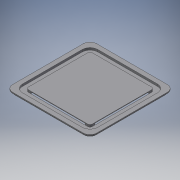
# Autodesk Inventor part: NewLid
Saved by Autodesk Inventor 2017 (Build 210142000, 142)
## iProperties
Created: 2019-11-20
Part Number: NewLid
Material: Generic
Document SubType Name: Modeling
Designer: DDeGo
Density: 1 g/cm^3
Appearance: Default
Author: DDeGo
Autodesk Inventor part; units mm, degrees
ref_plane "YZ Plane" through (0, 0, 0) normal (1, 0, 0) x (0, 1, 0)
ref_plane "XZ Plane" through (0, 0, 0) normal (0, 1, 0) x (-1, 0, 0)
ref_plane "XY Plane" through (0, 0, 0) normal (0, 0, 1) x (1, 0, 0)
sketch "Sketch1" plane through (0, 0, 0) normal (0, 0, 1) x (1, 0, 0)
  arc A0 (-15, -160) -> (0, -175) centre (0, -160) ccw
  line L0 (0, 15) -> (160, 15)
  line L1 (175, 0) -> (175, -160)
  line L2 (160, -175) -> (0, -175)
  line L3 (-15, -160) -> (-15, 0)
  arc A1 (0, 15) -> (-15, 0) centre (0, 0) ccw
  arc A2 (160, -175) -> (175, -160) centre (160, -160) ccw
  arc A3 (175, 0) -> (160, 15) centre (160, 0) ccw
  point P0 (-15, 15)
  dimension "d0" = 190
  dimension "d1" = 190
  dimension "d2" = 15
  constraints: 8 end point, 8 point on circle, 8 tangent, 4 centre point, 3 equal radius, 2 coincident, 2 parallel, 2 point on line, 1 horizontal, 1 perpendicular
  measures "d0" distance between parallel lines of L2 L0
  measures "d1" distance between parallel lines of L3 L1
  measures "d2" radius of A3
extrude "Extrusion1" add sketch "Sketch1" along normal blind 6.35
sketch "Sketch2" plane through (0, 0, 6.35) normal (0, 0, 1) x (1, 0, 0)
  line L0 (-15, 0) -> (-15, -160) projected
  arc A0 (-15, -160) -> (0, -175) centre (0, -160) ccw projected
  line L1 (0, -175) -> (160, -175) projected
  arc A1 (160, -175) -> (175, -160) centre (160, -160) ccw projected
  line L2 (175, -160) -> (175, 0) projected
  arc A2 (175, 0) -> (160, 15) centre (160, 0) ccw projected
  line L3 (160, 15) -> (0, 15) projected
  arc A3 (0, 15) -> (-15, 0) centre (0, 0) ccw projected
  line L4 (0, 0) -> (160, -160) construction
  line L5 (147.3, -152.3) -> (12.7, -152.3)
  line L6 (7.7, -147.3) -> (7.7, -12.7)
  line L7 (12.7, -7.7) -> (147.3, -7.7)
  line L8 (152.3, -12.7) -> (152.3, -147.3)
  line L9 (152.3, -152.3) -> (7.7, -7.7) construction
  line L10 (7.7, -152.3) -> (152.3, -7.7) construction
  arc A4 (12.7, -7.7) -> (7.7, -12.7) centre (12.7, -12.7) ccw
  arc A5 (152.3, -12.7) -> (147.3, -7.7) centre (147.3, -12.7) ccw
  arc A6 (147.3, -152.3) -> (152.3, -147.3) centre (147.3, -147.3) ccw
  arc A7 (7.7, -147.3) -> (12.7, -152.3) centre (12.7, -147.3) ccw
  line L11 (147.3, 5) -> (12.7, 5)
  arc A8 (12.7, 5) -> (-5, -12.7) centre (12.7, -12.7) ccw
  line L12 (-5, -12.7) -> (-5, -147.3)
  arc A9 (-5, -147.3) -> (12.7, -165) centre (12.7, -147.3) ccw
  line L13 (12.7, -165) -> (147.3, -165)
  arc A10 (147.3, -165) -> (165, -147.3) centre (147.3, -147.3) ccw
  line L14 (165, -147.3) -> (165, -12.7)
  arc A11 (165, -12.7) -> (147.3, 5) centre (147.3, -12.7) ccw
  point P0 (80, -80)
  dimension "d7" = 5
  dimension "d8" = 12.7
  dimension "d9" = 10
  constraints: 22 end point, 16 point on circle, 9 point on line, 8 centre point, 8 tangent, 4 parallel, 3 equal radius, 3 midpoint, 2 perpendicular, 1 horizontal, 7 other
  measures "d7" radius of A4
  measures "d8" distance between parallel lines of L7 L11
  measures "d9" distance between parallel lines of L2 L14
extrude "Extrusion2" cut sketch "Sketch2" against normal blind 5 contours A11 L14 A10 L13 A9 L12 A8 L11
sketch "Sketch3" plane through (0, 0, 0) normal (0, 0, -1) x (-1, 0, 0)
  line L0 (-140, -10.675) -> (-20, -10.675) construction
  line L1 (-147.3, -7.7) -> (-12.7, -7.7) projected
  line L2 (-140, -13.85) -> (-20, -13.85)
  line L3 (-20, -7.5) -> (-140, -7.5)
  arc A0 (-140, -7.5) -> (-140, -13.85) centre (-140, -10.675) ccw
  arc A1 (-20, -13.85) -> (-20, -7.5) centre (-20, -10.675) ccw
  line L4 (15, -160) -> (15, 0) projected
  line L5 (-175, 0) -> (-175, -160) projected
  arc A2 (-160, 15) -> (-175, 0) centre (-160, 0) ccw projected
  arc A3 (0, -175) -> (15, -160) centre (0, -160) ccw projected
  line L6 (-160, 0) -> (0, -160) construction
  circle A4 centre (-80, -80) radius 16.0572 construction
  arc A5 (-152.5, -140) -> (-146.15, -140) centre (-149.325, -140) ccw
  line L7 (-152.5, -20) -> (-152.5, -140)
  line L8 (-146.15, -140) -> (-146.15, -20)
  arc A6 (-146.15, -20) -> (-152.5, -20) centre (-149.325, -20) ccw
  line L9 (-149.325, -140) -> (-149.325, -20) construction
  arc A7 (-20, -152.5) -> (-20, -146.15) centre (-20, -149.325) ccw
  line L10 (-140, -152.5) -> (-20, -152.5)
  line L11 (-20, -146.15) -> (-140, -146.15)
  arc A8 (-140, -146.15) -> (-140, -152.5) centre (-140, -149.325) ccw
  line L12 (-20, -149.325) -> (-140, -149.325) construction
  arc A9 (-7.5, -20) -> (-13.85, -20) centre (-10.675, -20) ccw
  line L13 (-7.5, -140) -> (-7.5, -20)
  line L14 (-13.85, -20) -> (-13.85, -140)
  arc A10 (-13.85, -140) -> (-7.5, -140) centre (-10.675, -140) ccw
  line L15 (-10.675, -20) -> (-10.675, -140) construction
  point P0 (0, 0)
  point P1 (-80, -10.675)
  point P2 (-149.325, -80)
  point P3 (-80, -149.325)
  point P4 (-10.675, -80)
  dimension "d12" = 6.35
  dimension "d13" = 0.2
  dimension "d14" = 35
  dimension "d15" = 35
  dimension "d18" = 360
  constraints: 34 end point, 16 point on circle, 9 centre point, 4 tangent, 2 midpoint, 2 parallel, 49 other
  measures "d12" distance between parallel lines of L2 L3
  measures "d13" distance between parallel lines of L3 L1
  measures "d14" distance from line of L4 L0.end
  measures "d15" distance from line of L5 L0.start
extrude "Extrusion3" cut sketch "Sketch3" against normal blind 5
sketch "Sketch4" plane through (0, 0, 0) normal (0, 0, -1) x (-1, 0, 0)
  arc A0 (0, -175) -> (15, -160) centre (0, -160) ccw projected
  arc A1 (-160, 15) -> (-175, 0) centre (-160, 0) ccw projected
  line L0 (0, -160) -> (-160, 0) construction
  line L1 (-2, 11.5) -> (-158, 11.5)
  line L2 (-171.5, -2) -> (-171.5, -158)
  line L3 (-158, -171.5) -> (-2, -171.5)
  line L4 (11.5, -158) -> (11.5, -2)
  line L5 (11.5, 11.5) -> (-171.5, -171.5) construction
  line L6 (-171.5, 11.5) -> (11.5, -171.5) construction
  arc A2 (-2, -171.5) -> (11.5, -158) centre (-2, -158) ccw
  arc A3 (-171.5, -158) -> (-158, -171.5) centre (-158, -158) ccw
  arc A4 (-158, 11.5) -> (-171.5, -2) centre (-158, -2) ccw
  arc A5 (11.5, -2) -> (-2, 11.5) centre (-2, -2) ccw
  arc A6 (-20, -152.5) -> (-20, -146.15) centre (-20, -149.325) ccw projected
  line L7 (-20, -152.5) -> (-140, -152.5) projected
  arc A7 (-140, -146.15) -> (-140, -152.5) centre (-140, -149.325) ccw projected
  line L8 (-140, -146.15) -> (-20, -146.15) projected
  arc A8 (-20, -13.85) -> (-20, -7.5) centre (-20, -10.675) ccw projected
  line L9 (-20, -13.85) -> (-140, -13.85) projected
  arc A9 (-140, -7.5) -> (-140, -13.85) centre (-140, -10.675) ccw projected
  line L10 (-140, -7.5) -> (-20, -7.5) projected
  arc A10 (-152.5, -140) -> (-146.15, -140) centre (-149.325, -140) ccw projected
  line L11 (-152.5, -140) -> (-152.5, -20) projected
  arc A11 (-146.15, -20) -> (-152.5, -20) centre (-149.325, -20) ccw projected
  line L12 (-146.15, -20) -> (-146.15, -140) projected
  arc A12 (-7.5, -20) -> (-13.85, -20) centre (-10.675, -20) ccw projected
  line L13 (-7.5, -20) -> (-7.5, -140) projected
  arc A13 (-13.85, -140) -> (-7.5, -140) centre (-10.675, -140) ccw projected
  line L14 (-13.85, -140) -> (-13.85, -20) projected
  line L15 (15, -160) -> (15, 0) projected
  arc A14 (15, 0) -> (0, 15) centre (0, 0) ccw projected
  line L16 (0, 15) -> (-160, 15) projected
  arc A15 (-160, 15) -> (-175, 0) centre (-160, 0) ccw projected
  line L17 (-175, 0) -> (-175, -160) projected
  arc A16 (-175, -160) -> (-160, -175) centre (-160, -160) ccw projected
  line L18 (-160, -175) -> (0, -175) projected
  arc A17 (0, -175) -> (15, -160) centre (0, -160) ccw projected
  point P0 (-80, -80)
  dimension "d22" = 183
  dimension "d23" = 183
  dimension "d24" = 13.5
  constraints: 14 end point, 8 point on circle, 8 point on line, 8 tangent, 4 centre point, 3 equal radius, 3 midpoint, 2 parallel, 1 horizontal, 1 perpendicular
  measures "d22" distance of L5.end L6.end
  measures "d23" distance of L6.start L5.end
  measures "d24" radius of A2
extrude "Extrusion4" cut sketch "Sketch4" against normal blind 4 contours L18 A16 L17 A1 L16 A14 L15 A0
equation "\"d14\" = d15"
body "Solid1"
